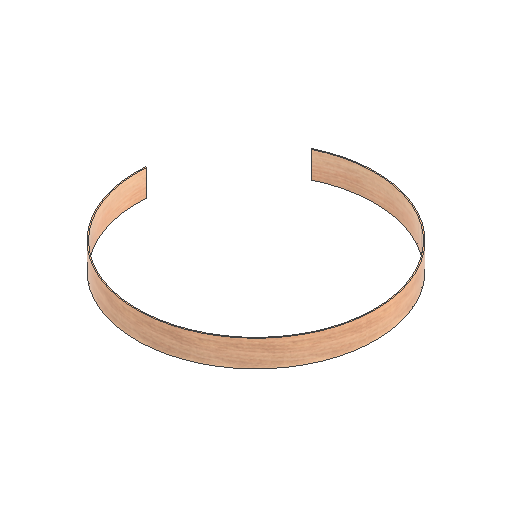
# Autodesk Inventor part: Edge Band - Disk A Inner
Saved by Autodesk Inventor 2021 (Build 250183000, 183)
## iProperties
Created: 2020-05-12
Part Number: Edge Band - Disk A Inner
Material: Wood (Birch)
Document SubType Name: Modeling
Designer: Dan Wikman
Density: 0.55 g/cm^3
Appearance: Birch - Natural Polished
Mass: 516.051 g
Surface Area: 4887.72 cm^2
Volume: 938.274 cm^3
Author: Dan Wikman
Autodesk Inventor part; units mm, degrees
ref_plane "YZ Plane" through (0, 0, 0) normal (1, 0, 0) x (0, 1, 0)
ref_plane "XZ Plane" through (0, 0, 0) normal (0, 1, 0) x (-1, 0, 0)
ref_plane "XY Plane" through (0, 0, 0) normal (0, 0, 1) x (1, 0, 0)
sketch "Sketch1" plane through (0, 0, 0) normal (0, 1, 0) x (-1, 0, 0)
  circle A0 centre (0, 0) radius 450
  circle A1 centre (0, 0) radius 446
  dimension "d0" = 900
  dimension "d1" = 892
  constraints: 2 centre point, 2 coincident
  measures "d0" diameter of A0
  measures "d1" diameter of A1
extrude "Extrusion1" add sketch "Sketch1" along normal blind 100
sketch "Sketch2" plane through (0, 0, 0) normal (0, -1, 0) x (1, 0, 0)
  line L0 (-195.5443, -404.3283) -> (-647.1656, -801.922) projected
  line L1 (-983.2067, -310.7574) -> (-448.704, -34.1743) projected
  circle A0 centre (0, 0) radius 450 projected
  circle A1 centre (0, 0) radius 446 projected
  line L2 (-192.9926, -402.0819) -> (-196.2516, -404.951)
  line L3 (-444.838, -32.1738) -> (-448.704, -34.1743)
  point P0 (-448.7006, -34.1726)
  constraints: 4 end point, 3 point on line, 2 point on circle, 1 collinear, 2 other
extrude "Extrusion2" cut sketch "Sketch2" against normal blind 100 contours L0 A0 L3 A1 L2 picked at (-445.1017, -42.5508)
body "Solid1"
